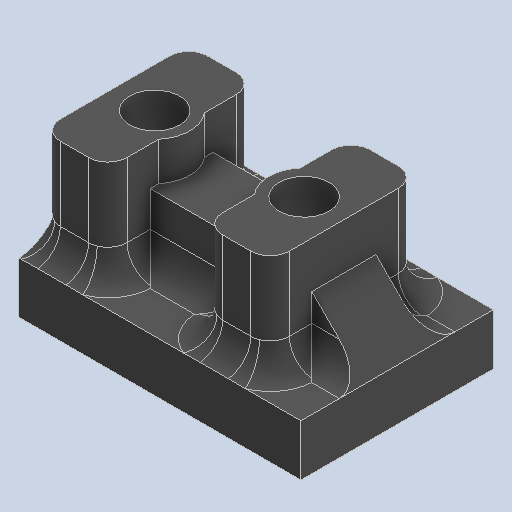
# Autodesk Inventor part: Primer inserto
Saved by Autodesk Inventor 2026 (Build 300175050, 175E)
## iProperties
Created: 2025-09-26
Part Number: Primer inserto
Material: Plastico PETG
Document SubType Name: Modeling
Designer: bello
Density: 1.27 g/cm^3
Appearance: Genérico
Author: bello
Autodesk Inventor part; units mm, degrees
ref_plane "YZ Plane" through (0, 0, 0) normal (1, 0, 0) x (0, 1, 0)
ref_plane "XZ Plane" through (0, 0, 0) normal (0, 1, 0) x (-1, 0, 0)
sketch "Boceto1" plane through (0, 0, 0) normal (0, 1, 0) x (-1, 0, 0)
  line L0 (0, 0) -> (-44, 0)
  line L1 (-44, 0) -> (-44, -30)
  line L2 (-44, -30) -> (0, -30)
  line L3 (0, -30) -> (0, 0)
  dimension "d0" = 30
  dimension "d1" = 44
  constraints: 8 end point, 2 parallel, 1 horizontal, 1 perpendicular
  measures "d0" distance of L2.end L0.start
  measures "d1" distance of L1.end L2.end
extrude "Extrusión1" add sketch "Boceto1" along normal blind 8
sketch "Boceto2" plane through (0, 8, 0) normal (0, 1, 0) x (1, 0, 0)
  line L0 (-5.2329, 15) -> (48.4559, 15)
  line L1 (3, 26.5) -> (7.4, 26.5)
  line L2 (10.4, 23.5) -> (10.4, 6.5)
  line L3 (7.4, 3.5) -> (3, 3.5)
  line L4 (0, 6.5) -> (0, 15)
  line L5 (0, 30) -> (0, 0) projected
  line L6 (0, 15) -> (0, 23.5)
  arc A0 (0, 6.5) -> (3, 3.5) centre (3, 6.5) ccw
  arc A1 (3, 26.5) -> (0, 23.5) centre (3, 23.5) ccw
  arc A2 (10.4, 23.5) -> (7.4, 26.5) centre (7.4, 23.5) ccw
  arc A3 (7.4, 3.5) -> (10.4, 6.5) centre (7.4, 6.5) ccw
  line L7 (10.4, 15) -> (25.3, 15)
  line L8 (25.3, 15) -> (25.3, 19.9)
  line L9 (25.3, 19.9) -> (10.4, 19.9)
  line L10 (10.4, 19.9) -> (10.4, 15)
  line L11 (10.4, 15) -> (25.3, 15)
  line L12 (25.3, 15) -> (25.3, 10.1)
  line L13 (25.3, 10.1) -> (10.4, 10.1)
  line L14 (10.4, 10.1) -> (10.4, 15)
  line L15 (17.85, -3.2018) -> (17.85, 35.6428)
  line L16 (32.7, 26.5) -> (28.3, 26.5)
  line L17 (25.3, 23.5) -> (25.3, 6.5)
  line L18 (28.3, 3.5) -> (32.7, 3.5)
  line L19 (35.7, 6.5) -> (35.7, 15)
  line L20 (35.7, 15) -> (35.7, 23.5)
  arc A4 (32.7, 3.5) -> (35.7, 6.5) centre (32.7, 6.5) ccw
  arc A5 (35.7, 23.5) -> (32.7, 26.5) centre (32.7, 23.5) ccw
  arc A6 (28.3, 26.5) -> (25.3, 23.5) centre (28.3, 23.5) ccw
  arc A7 (25.3, 6.5) -> (28.3, 3.5) centre (28.3, 6.5) ccw
  line L21 (25.3, 19.9) -> (25.3, 15)
  line L22 (25.3, 10.1) -> (25.3, 15)
  point P0 (0, 26.5)
  point P1 (10.4, 26.5)
  point P2 (0, 3.5)
  point P3 (40.9329, 15)
  point P4 (35.7, 26.5)
  point P5 (25.3, 26.5)
  point P6 (35.7, 3.5)
  dimension "d5" = 11.5
  dimension "d6" = 11.5
  dimension "d7" = 10.4
  dimension "d8" = 3
  dimension "d9" = 14.9
  dimension "d10" = 4.9
  dimension "d11" = 4.9
  dimension "d12" = 9.8
  dimension "d13" = 35.7
  constraints: 44 end point, 17 symmetric about line, 16 point on circle, 13 point on line, 8 centre point, 8 tangent, 5 equal length, 5 horizontal, 4 perpendicular, 3 equal radius, 2 midpoint, 1 vertical, 4 other
  measures "d5" distance of point (0, 3.5) L4.end
  measures "d6" distance of L4.end point (0, 26.5)
  measures "d7" distance of point (0, 26.5) point (10.4, 26.5)
  measures "d8" radius of A0
  measures "d9" distance of L8.end L9.end
  measures "d10" distance of L9.end L7.start
  measures "d11" distance of L13.end L7.start
  measures "d12" distance between parallel lines of L13 L9
  measures "d13" distance between parallel lines of L20 L5
extrude "Extrusión2" add sketch "Boceto2" along normal blind 15.5
sketch "Boceto3" plane through (0, 23.5, 0) normal (0, 1, 0) x (1, 0, 0)
  circle A0 centre (6.2, 15) radius 5.5
  circle A1 centre (29.5, 15) radius 5.5
  line L0 (0, 23.5) -> (0, 6.5) projected
  line L1 (35.7, 6.5) -> (35.7, 23.5) projected
  line L2 (10.4, 10.1) -> (10.4, 6.5) projected
  line L3 (10.4, 10.1) -> (10.4, 11.4489)
  line L4 (10.4, 19.9) -> (25.3, 19.9) projected
  line L5 (10.4, 18.5511) -> (10.4, 19.9)
  line L6 (10.4, 10.1) -> (25.3, 10.1) projected
  line L7 (25.3, 11.4489) -> (25.3, 10.1)
  line L8 (25.3, 18.5511) -> (25.3, 19.9)
  line L9 (25.3, 19.9) -> (10.4, 19.9)
  point P0 (0, 0)
  dimension "d16" = 6.2
  dimension "d17" = 6.2
  dimension "d18" = 11
  dimension "d19" = 11
  dimension "d26" = 23.3
  constraints: 10 end point, 4 point on circle, 3 perpendicular, 2 centre point, 2 point on line, 1 collinear
  measures "d16" distance from line of L0 A0.centre
  measures "d17" distance from line of L1 A1.centre
  measures "d18" diameter of A0
  measures "d19" diameter of A1
  measures "d26" distance of A1.centre A0.centre
extrude "Extrusión3" cut sketch "Boceto3" against normal blind 6 contours A0 L5 L4 L8 A1 L7 L6 L3
sketch "Boceto4" plane through (0, 23.5, 0) normal (0, 1, 0) x (1, 0, 0)
  arc A0 (10.4, 11.4489) -> (10.4, 18.5511) centre (6.2, 15) ccw projected
  circle A1 centre (6.2, 15) radius 3.9
  arc A2 (25.3, 18.5511) -> (25.3, 11.4489) centre (29.5, 15) ccw projected
  circle A3 centre (29.5, 15) radius 3.9
  point P0 (0, 0)
  dimension "d22" = 7.8
  dimension "d23" = 7.8
  constraints: 2 centre point, 2 coincident
  measures "d22" diameter of A1
  measures "d23" diameter of A3
extrude "Extrusión4" cut sketch "Boceto4" against normal blind 15.5
sketch "Boceto5" plane through (6.2, 8, -15) normal (0, 1, 0) x (1, 0, 0)
  circle A0 centre (0, 0) radius 3.9 projected
  circle A1 centre (0, 0) radius 1.25
  circle A2 centre (23.3, 0) radius 3.9 projected
  circle A3 centre (23.3, 0) radius 1.25
  point P0 (-6.2, -15)
  dimension "d27" = 2.5
  dimension "d28" = 2.5
  constraints: 2 centre point, 2 coincident
  measures "d27" diameter of A1
  measures "d28" diameter of A3
extrude "Extrusión5" cut sketch "Boceto5" against normal blind 8 contours A1 | A3
ref_plane "Plano de trabajo1" through (0, 0, -15) normal (0, 0, 1) x (1, 0, 0)
sketch "Boceto6" plane through (0, 0, -15) normal (0, 0, 1) x (1, 0, 0)
  line L0 (0, 8) -> (44, 8) projected
  line L1 (35.7, 8) -> (35.7, 23.5) projected
  line L2 (44, 8) -> (35.7, 8)
  line L3 (35.7, 8) -> (35.7, 16.3)
  line L4 (35.7, 16.3) -> (44, 8)
  point P0 (0, 0)
  dimension "d32" = 8.3
  constraints: 6 end point, 1 horizontal, 1 perpendicular
  measures "d32" distance of L1.start L3.end
extrude "Extrusión6" add sketch "Boceto6" along normal mid plane 10
fillet "Empalme2" radius 4 22 edges at (17.85, 8, -10.1) (25.3, 8, -8.3) (30.5, 8, -3.5) (34.8213, 8, -4.3787) (35.7, 8, -8.25) (26.1787, 8, -4.3787) (39.85, 8, -10) (34.8213, 8, -25.6213) (30.5, 8, -26.5) (26.1787, 8, -25.6213) (25.3, 8, -21.7) (35.7, 8, -21.75) (39.85, 8, -20) (17.85, 8, -19.9) (10.4, 8, -21.7) (5.2, 8, -26.5) (0.8787, 8, -25.6213) (9.5213, 8, -25.6213) (5.2, 8, -3.5) (0.8787, 8, -4.3787) (10.4, 8, -8.3) (9.5213, 8, -4.3787)
